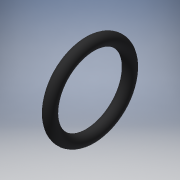
# Autodesk Inventor part: 9396K27 Silicone O-Ring
Saved by Autodesk Inventor 2019.4 (Build 234330000, 330)
## iProperties
Created: 2012-06-04
Part Number: 9396K27 Silicone O-Ring
Material: Rubber, Silicone
Document SubType Name: Modeling
Designer: ding42
Mass: 0.383382 g
Surface Area: 4.68933 cm^2
Volume: 0.306705 cm^3
Density: 1.25 g/cm^3
Description: Dash Number 114
Appearance: Rubber - Black
Author: ding42
Autodesk Inventor part; units mm, degrees
ref_plane "YZ Plane" through (0, 0, 0) normal (1, 0, 0) x (0, 1, 0)
ref_plane "XZ Plane" through (0, 0, 0) normal (0, 1, 0) x (-1, 0, 0)
ref_plane "XY Plane" through (0, 0, 0) normal (0, 0, 1) x (1, 0, 0)
sketch "Sketch1" plane through (0, 0, 0) normal (0, 0, 1) x (1, 0, 0)
  circle A0 centre (0, 0) radius 1.3081
  dimension "d0" = 2.6162
  constraints: 1 centre point, 1 coincident
  measures "d0" diameter of A0
sketch "Sketch2" plane through (0, 0, 0) normal (1, 0, 0) x (0, 1, 0)
  circle A0 centre (9.0805, 0) radius 7.7724
  line L0 (1.3081, 0) -> (-1.3081, 0) projected
  point P0 (0, 0)
  dimension "d1" = 15.5448
  constraints: 1 horizontal alignment, 2 other
sweep "Sweep1" add profiles "Sketch1" path "Sketch2" path curves A0
body "Solid1"
